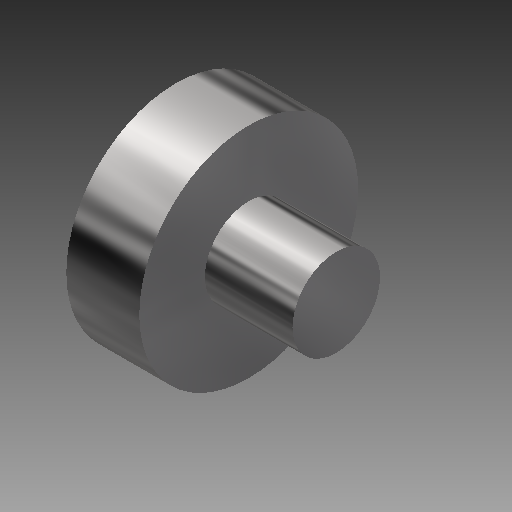
# Autodesk Inventor part: 404-02
Saved by Autodesk Inventor 2019 (Build 230136000, 136)
## iProperties
Company: Autodesk Inc.
Created: 2017-06-27
Part Number: 404-02
Material: Steel, Mild
Document SubType Name: Modeling
Designer: Autodesk Inc.
Mass: 0.129184 g
Surface Area: 0.438841 cm^2
Volume: 0.0164565 cm^3
Density: 7.85 g/cm^3
Appearance: Semi-Polished
Author: Inventor
Autodesk Inventor part; units mm, degrees
ref_plane "YZ Plane" through (0, 0, 0) normal (1, 0, 0) x (0, 1, 0)
ref_plane "XZ Plane" through (0, 0, 0) normal (0, 1, 0) x (-1, 0, 0)
ref_plane "XY Plane" through (0, 0, 0) normal (0, 0, 1) x (1, 0, 0)
sketch "Sketch1" plane through (0, 0, 0) normal (0, 0, 1) x (1, 0, 0)
  line L0 (0, 0) -> (1.25, 0)
  line L1 (1.25, 0) -> (1.25, 1.875)
  line L2 (1.25, 1.875) -> (0, 1.875)
  line L3 (0, 1.875) -> (0, 0)
  line L4 (1.25, 0) -> (2.75, 0)
  line L5 (2.75, 0) -> (2.75, 0.75)
  line L6 (2.75, 0.75) -> (1.25, 0.75)
  line L7 (1.25, 0.75) -> (1.25, 0)
  dimension "d0" = 1.25
  dimension "d1" = 2.75
  dimension "d2" = 1.5
  dimension "d3" = 3.75
  constraints: 16 end point, 4 parallel, 2 horizontal, 2 perpendicular
  measures "d0" distance of L1.end L2.end
  measures "d1" distance between parallel lines of L5 L3
  measures "d2" diameter of L6 L4
  measures "d3" diameter of L2 L4
revolve "Revolution1" add sketch "Sketch1" angle 360 about axis through (0, 0, 0) along (1, 0, 0)
body "Solid1"
